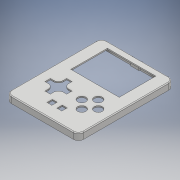
# Autodesk Inventor part: CaseOutline
Saved by Autodesk Inventor 2017 SP1 (Build 210196100, 196)
## iProperties
Created: 2017-08-23
Part Number: CaseOutline
Material: Generic
Document SubType Name: Modeling
Designer: Groguard
Density: 1 g/cm^3
Appearance: Default
Author: Groguard
Autodesk Inventor part; units mm, degrees
ref_plane "YZ Plane" through (0, 0, 0) normal (1, 0, 0) x (0, 1, 0)
ref_plane "XZ Plane" through (0, 0, 0) normal (0, 1, 0) x (-1, 0, 0)
ref_plane "XY Plane" through (0, 0, 0) normal (0, 0, 1) x (1, 0, 0)
sketch "Sketch1" plane through (0, 0, 0) normal (0, 0, 1) x (1, 0, 0)
  line L0 (3.4142, 110) -> (35, 110)
  line L1 (47, 110) -> (78.5858, 110)
  arc A0 (82, 106.5858) -> (78.5858, 110) centre (78.5858, 106.5858) ccw
  arc A1 (47, 110) -> (46, 109) centre (47, 109) ccw
  arc A2 (36, 109) -> (35, 110) centre (35, 109) ccw
  line L2 (36, 109) -> (46, 109)
  arc A3 (3.4142, 110) -> (0, 106.5858) centre (3.4142, 106.5858) ccw
  line L3 (0, 106.5858) -> (0, 3.4142)
  arc A4 (0, 3.4142) -> (3.4142, 0) centre (3.4142, 3.4142) ccw
  arc A5 (78.5858, 0) -> (82, 3.4142) centre (78.5858, 3.4142) ccw
  line L4 (82, 3.4142) -> (82, 106.5858)
  line L5 (3.4142, 0) -> (78.5858, 0)
  line L6 (-3, 3.4142) -> (-3, 106.5858)
  arc A6 (3.4142, 113) -> (-3, 106.5858) centre (3.4142, 106.5858) ccw
  line L7 (3.4142, 113) -> (35, 113)
  arc A7 (37.6458, 112) -> (35, 113) centre (35, 109) ccw
  line L8 (37.6458, 112) -> (44.3542, 112)
  arc A8 (47, 113) -> (44.3542, 112) centre (47, 109) ccw
  line L9 (47, 113) -> (78.5858, 113)
  arc A9 (85, 106.5858) -> (78.5858, 113) centre (78.5858, 106.5858) ccw
  line L10 (85, 106.5858) -> (85, 3.4142)
  arc A10 (78.5858, -3) -> (85, 3.4142) centre (78.5858, 3.4142) ccw
  line L11 (78.5858, -3) -> (3.4142, -3)
  arc A11 (-3, 3.4142) -> (3.4142, -3) centre (3.4142, 3.4142) ccw
  arc A12 (70.4, 61.0119) -> (70.4, 61.0881) centre (70.4, 61.05) ccw
  arc A13 (11.6, 61.0881) -> (11.6, 61.0119) centre (11.6, 61.05) ccw
  line L12 (70.4, 61.05) -> (70.4, 105.55)
  arc A14 (70.4381, 105.55) -> (70.3619, 105.55) centre (70.4, 105.55) ccw
  arc A15 (70.3619, 61.05) -> (70.4381, 61.05) centre (70.4, 61.05) ccw
  arc A16 (11.6, 105.5881) -> (11.6, 105.5119) centre (11.6, 105.55) ccw
  arc A17 (70.4, 105.5119) -> (70.4, 105.5881) centre (70.4, 105.55) ccw
  line L13 (11.6, 105.55) -> (11.6, 61.05)
  arc A18 (11.5619, 61.05) -> (11.6381, 61.05) centre (11.6, 61.05) ccw
  arc A19 (11.6381, 105.55) -> (11.5619, 105.55) centre (11.6, 105.55) ccw
  line L14 (11.6, 61.05) -> (70.4, 61.05)
  arc A20 (30.1856, 85.7097) -> (30.4452, 85.4501) centre (30.4452, 85.7097) ccw
  arc A21 (30.211, 85.7097) -> (30.1602, 85.7097) centre (30.1856, 85.7097) ccw
  arc A22 (30.4452, 85.4247) -> (30.4452, 85.4755) centre (30.4452, 85.4501) ccw
  line L15 (30.1856, 85.7097) -> (30.1856, 85.7746)
  arc A23 (30.211, 85.7746) -> (30.1602, 85.7746) centre (30.1856, 85.7746) ccw
  arc A24 (30.1602, 85.7097) -> (30.211, 85.7097) centre (30.1856, 85.7097) ccw
  arc A25 (30.8347, 85.7746) -> (30.1856, 85.7746) centre (30.5102, 85.7746) ccw
  arc A26 (30.8093, 85.7746) -> (30.8601, 85.7746) centre (30.8347, 85.7746) ccw
  arc A27 (30.1602, 85.7746) -> (30.211, 85.7746) centre (30.1856, 85.7746) ccw
  line L16 (30.8347, 85.7746) -> (30.8347, 85.4501)
  arc A28 (30.8093, 85.4501) -> (30.8601, 85.4501) centre (30.8347, 85.4501) ccw
  arc A29 (30.8601, 85.7746) -> (30.8093, 85.7746) centre (30.8347, 85.7746) ccw
  arc A30 (30.3154, 84.9308) -> (30.8347, 85.4501) centre (30.3154, 85.4501) ccw
  arc A31 (30.3154, 84.9562) -> (30.3154, 84.9054) centre (30.3154, 84.9308) ccw
  arc A32 (30.8601, 85.4501) -> (30.8093, 85.4501) centre (30.8347, 85.4501) ccw
  line L17 (31.3286, 84.9308) -> (31.6531, 84.9308)
  arc A33 (31.6531, 84.9054) -> (31.6531, 84.9562) centre (31.6531, 84.9308) ccw
  arc A34 (31.3286, 84.9562) -> (31.3286, 84.9054) centre (31.3286, 84.9308) ccw
  arc A35 (31.6531, 84.9308) -> (31.6531, 85.5799) centre (31.6531, 85.2553) ccw
  arc A36 (31.6531, 84.9562) -> (31.6531, 84.9054) centre (31.6531, 84.9308) ccw
  arc A37 (31.6531, 85.6053) -> (31.6531, 85.5545) centre (31.6531, 85.5799) ccw
  line L18 (31.3286, 86.0992) -> (31.7181, 86.0992)
  arc A38 (31.7181, 86.0738) -> (31.7181, 86.1246) centre (31.7181, 86.0992) ccw
  arc A39 (31.3286, 86.1246) -> (31.3286, 86.0738) centre (31.3286, 86.0992) ccw
  arc A40 (31.7181, 85.5799) -> (31.7181, 86.0992) centre (31.7181, 85.8396) ccw
  arc A41 (31.7181, 85.6053) -> (31.7181, 85.5545) centre (31.7181, 85.5799) ccw
  arc A42 (31.7181, 86.1246) -> (31.7181, 86.0738) centre (31.7181, 86.0992) ccw
  line L19 (31.7181, 85.5799) -> (31.4584, 85.5799)
  arc A43 (31.4584, 85.6053) -> (31.4584, 85.5545) centre (31.4584, 85.5799) ccw
  arc A44 (31.7181, 85.5545) -> (31.7181, 85.6053) centre (31.7181, 85.5799) ccw
  line L20 (32.7312, 86.0992) -> (32.4716, 85.1904)
  arc A45 (32.4472, 85.1974) -> (32.496, 85.1835) centre (32.4716, 85.1904) ccw
  arc A46 (32.7557, 86.0922) -> (32.7068, 86.1062) centre (32.7313, 86.0992) ccw
  line L21 (32.4716, 85.1904) -> (33.1207, 85.1904)
  arc A47 (33.1207, 85.165) -> (33.1207, 85.2158) centre (33.1207, 85.1904) ccw
  arc A48 (32.4716, 85.2158) -> (32.4716, 85.165) centre (32.4716, 85.1904) ccw
  line L22 (32.926, 85.4501) -> (32.926, 84.9308)
  arc A49 (32.9006, 84.9308) -> (32.9514, 84.9308) centre (32.926, 84.9308) ccw
  arc A50 (32.9514, 85.4501) -> (32.9006, 85.4501) centre (32.926, 85.4501) ccw
  line L23 (33.6146, 85.8396) -> (33.9391, 86.0992)
  arc A51 (33.955, 86.0794) -> (33.9233, 86.119) centre (33.9391, 86.0992) ccw
  arc A52 (33.5987, 85.8594) -> (33.6304, 85.8197) centre (33.6146, 85.8396) ccw
  line L24 (33.9391, 86.0992) -> (33.9391, 84.9308)
  arc A53 (33.9137, 84.9308) -> (33.9645, 84.9308) centre (33.9391, 84.9308) ccw
  arc A54 (33.9645, 86.0992) -> (33.9137, 86.0992) centre (33.9391, 86.0992) ccw
  line L25 (33.6146, 84.9308) -> (34.2637, 84.9308)
  arc A55 (34.2637, 84.9054) -> (34.2637, 84.9562) centre (34.2637, 84.9308) ccw
  arc A56 (33.6146, 84.9562) -> (33.6146, 84.9054) centre (33.6146, 84.9308) ccw
  line L26 (34.7689, 85.3852) -> (35.5478, 85.3852)
  arc A57 (35.5478, 85.3598) -> (35.5478, 85.4106) centre (35.5478, 85.3852) ccw
  arc A58 (34.7689, 85.4106) -> (34.7689, 85.3598) centre (34.7689, 85.3852) ccw
  arc A59 (36.7021, 85.8071) -> (36.41, 86.0992) centre (36.41, 85.8071) ccw
  arc A60 (36.6767, 85.8071) -> (36.7275, 85.8071) centre (36.7021, 85.8071) ccw
  arc A61 (36.41, 86.1246) -> (36.41, 86.0738) centre (36.41, 86.0992) ccw
  arc A62 (36.41, 86.0992) -> (36.053, 85.8396) centre (36.41, 85.724) ccw
  arc A63 (36.41, 86.0738) -> (36.41, 86.1246) centre (36.41, 86.0992) ccw
  arc A64 (36.0288, 85.8474) -> (36.0771, 85.8317) centre (36.0529, 85.8396) ccw
  arc A65 (36.6047, 85.5799) -> (36.7021, 85.8071) centre (36.3884, 85.8071) ccw
  arc A66 (36.5872, 85.5983) -> (36.6222, 85.5615) centre (36.6047, 85.5799) ccw
  arc A67 (36.7275, 85.8071) -> (36.6767, 85.8071) centre (36.7021, 85.8071) ccw
  line L27 (36.6047, 85.5799) -> (36.053, 84.9308)
  arc A68 (36.0336, 84.9473) -> (36.0723, 84.9143) centre (36.0529, 84.9308) ccw
  arc A69 (36.6241, 85.5635) -> (36.5854, 85.5964) centre (36.6047, 85.5799) ccw
  line L28 (36.053, 84.9308) -> (36.7021, 84.9308)
  arc A70 (36.7021, 84.9054) -> (36.7021, 84.9562) centre (36.7021, 84.9308) ccw
  arc A71 (36.053, 84.9562) -> (36.053, 84.9054) centre (36.053, 84.9308) ccw
  arc A72 (37.8451, 85.2554) -> (37.196, 85.2554) centre (37.5206, 85.2554) ccw
  arc A73 (37.8197, 85.2554) -> (37.8705, 85.2554) centre (37.8451, 85.2554) ccw
  arc A74 (37.1706, 85.2554) -> (37.2214, 85.2554) centre (37.196, 85.2554) ccw
  arc A75 (37.196, 85.2554) -> (37.8451, 85.2554) centre (37.5206, 85.2554) ccw
  arc A76 (37.2214, 85.2554) -> (37.1706, 85.2554) centre (37.196, 85.2554) ccw
  arc A77 (37.8705, 85.2554) -> (37.8197, 85.2554) centre (37.8451, 85.2554) ccw
  arc A78 (37.7802, 85.8396) -> (37.2609, 85.8396) centre (37.5206, 85.8396) ccw
  arc A79 (37.7548, 85.8396) -> (37.8056, 85.8396) centre (37.7802, 85.8396) ccw
  arc A80 (37.2355, 85.8396) -> (37.2863, 85.8396) centre (37.2609, 85.8396) ccw
  arc A81 (37.2609, 85.8396) -> (37.7802, 85.8396) centre (37.5206, 85.8396) ccw
  arc A82 (37.2863, 85.8396) -> (37.2355, 85.8396) centre (37.2609, 85.8396) ccw
  arc A83 (37.8056, 85.8396) -> (37.7548, 85.8396) centre (37.7802, 85.8396) ccw
  line L29 (50, 18.25) -> (50, 11.75)
  arc A84 (50.0508, 18.25) -> (49.9492, 18.25) centre (50, 18.25) ccw
  line L30 (50, 11.75) -> (44, 11.75)
  line L31 (44, 11.75) -> (44, 18.25)
  arc A85 (44.0508, 18.25) -> (43.9492, 18.25) centre (44, 18.25) ccw
  line L32 (44, 18.25) -> (50, 18.25)
  arc A86 (50, 18.1992) -> (50, 18.3008) centre (50, 18.25) ccw
  arc A87 (44, 18.3008) -> (44, 18.1992) centre (44, 18.25) ccw
  line L33 (38, 18.25) -> (38, 11.75)
  arc A88 (38.0508, 18.25) -> (37.9492, 18.25) centre (38, 18.25) ccw
  line L34 (38, 11.75) -> (32, 11.75)
  line L35 (32, 11.75) -> (32, 18.25)
  arc A89 (32.0508, 18.25) -> (31.9492, 18.25) centre (32, 18.25) ccw
  line L36 (32, 18.25) -> (38, 18.25)
  arc A90 (38, 18.1992) -> (38, 18.3008) centre (38, 18.25) ccw
  arc A91 (32, 18.3008) -> (32, 18.1992) centre (32, 18.25) ccw
  line L37 (3.96, 108.28) -> (73.16, 108.28)
  arc A92 (73.16, 108.2482) -> (73.16, 108.3118) centre (73.16, 108.28) ccw
  arc A93 (3.96, 108.3118) -> (3.96, 108.2482) centre (3.96, 108.28) ccw
  line L38 (73.16, 108.28) -> (73.16, 58.28)
  arc A94 (73.1282, 58.28) -> (73.1917, 58.28) centre (73.16, 58.28) ccw
  arc A95 (73.1917, 108.28) -> (73.1282, 108.28) centre (73.16, 108.28) ccw
  line L39 (73.16, 58.28) -> (3.96, 58.28)
  arc A96 (3.96, 58.3118) -> (3.96, 58.2482) centre (3.96, 58.28) ccw
  arc A97 (73.16, 58.2482) -> (73.16, 58.3118) centre (73.16, 58.28) ccw
  line L40 (3.96, 58.28) -> (3.96, 108.28)
  arc A98 (3.9918, 108.28) -> (3.9283, 108.28) centre (3.96, 108.28) ccw
  arc A99 (3.9283, 58.28) -> (3.9918, 58.28) centre (3.96, 58.28) ccw
  line L41 (20.6108, 93.6396) -> (20.9354, 93.8992)
  arc A100 (20.9512, 93.8794) -> (20.9195, 93.919) centre (20.9353, 93.8992) ccw
  arc A101 (20.5949, 93.6594) -> (20.6267, 93.6197) centre (20.6108, 93.6396) ccw
  line L42 (20.9354, 93.8992) -> (20.9354, 92.7308)
  arc A102 (20.91, 92.7308) -> (20.9608, 92.7308) centre (20.9354, 92.7308) ccw
  arc A103 (20.9608, 93.8992) -> (20.91, 93.8992) centre (20.9354, 93.8992) ccw
  line L43 (20.6108, 92.7308) -> (21.2599, 92.7308)
  arc A104 (21.2599, 92.7054) -> (21.2599, 92.7562) centre (21.2599, 92.7308) ccw
  arc A105 (20.6108, 92.7562) -> (20.6108, 92.7054) centre (20.6108, 92.7308) ccw
  line L44 (20.6108, 74.2396) -> (20.9354, 74.4992)
  arc A106 (20.9512, 74.4794) -> (20.9195, 74.519) centre (20.9353, 74.4992) ccw
  arc A107 (20.5949, 74.2594) -> (20.6267, 74.2197) centre (20.6108, 74.2396) ccw
  line L45 (20.9354, 74.4992) -> (20.9354, 73.3308)
  arc A108 (20.91, 73.3308) -> (20.9608, 73.3308) centre (20.9354, 73.3308) ccw
  arc A109 (20.9608, 74.4992) -> (20.91, 74.4992) centre (20.9354, 74.4992) ccw
  line L46 (20.6108, 73.3308) -> (21.2599, 73.3308)
  arc A110 (21.2599, 73.3054) -> (21.2599, 73.3562) centre (21.2599, 73.3308) ccw
  arc A111 (20.6108, 73.3562) -> (20.6108, 73.3054) centre (20.6108, 73.3308) ccw
  arc A112 (22.4029, 73.6554) -> (21.7538, 73.6554) centre (22.0784, 73.6554) ccw
  arc A113 (22.3775, 73.6554) -> (22.4283, 73.6554) centre (22.4029, 73.6554) ccw
  arc A114 (21.7284, 73.6554) -> (21.7792, 73.6554) centre (21.7538, 73.6554) ccw
  arc A115 (21.7538, 73.6554) -> (22.4029, 73.6554) centre (22.0784, 73.6554) ccw
  arc A116 (21.7792, 73.6554) -> (21.7284, 73.6554) centre (21.7538, 73.6554) ccw
  arc A117 (22.4283, 73.6554) -> (22.3775, 73.6554) centre (22.4029, 73.6554) ccw
  arc A118 (22.338, 74.2396) -> (21.8187, 74.2396) centre (22.0784, 74.2396) ccw
  arc A119 (22.3126, 74.2396) -> (22.3634, 74.2396) centre (22.338, 74.2396) ccw
  arc A120 (21.7933, 74.2396) -> (21.8441, 74.2396) centre (21.8187, 74.2396) ccw
  arc A121 (21.8187, 74.2396) -> (22.338, 74.2396) centre (22.0784, 74.2396) ccw
  arc A122 (21.8441, 74.2396) -> (21.7933, 74.2396) centre (21.8187, 74.2396) ccw
  arc A123 (22.3634, 74.2396) -> (22.3126, 74.2396) centre (22.338, 74.2396) ccw
  line L47 (28.6433, 84.9308) -> (28.6433, 85.7097)
  arc A124 (28.6687, 85.7097) -> (28.6179, 85.7097) centre (28.6433, 85.7097) ccw
  arc A125 (28.6179, 84.9308) -> (28.6687, 84.9308) centre (28.6433, 84.9308) ccw
  line L48 (28.6108, 86.0343) -> (28.6108, 86.0992)
  arc A126 (28.6362, 86.0992) -> (28.5854, 86.0992) centre (28.6108, 86.0992) ccw
  arc A127 (28.5854, 86.0343) -> (28.6362, 86.0343) centre (28.6108, 86.0343) ccw
  line L49 (28.6108, 86.0992) -> (28.6757, 86.0992)
  arc A128 (28.6757, 86.0738) -> (28.6757, 86.1246) centre (28.6757, 86.0992) ccw
  arc A129 (28.6108, 86.1246) -> (28.6108, 86.0738) centre (28.6108, 86.0992) ccw
  line L50 (28.6757, 86.0992) -> (28.6757, 86.0343)
  arc A130 (28.6503, 86.0343) -> (28.7011, 86.0343) centre (28.6757, 86.0343) ccw
  arc A131 (28.7011, 86.0992) -> (28.6503, 86.0992) centre (28.6757, 86.0992) ccw
  line L51 (28.6757, 86.0343) -> (28.6108, 86.0343)
  arc A132 (28.6108, 86.0597) -> (28.6108, 86.0089) centre (28.6108, 86.0343) ccw
  arc A133 (28.6757, 86.0089) -> (28.6757, 86.0597) centre (28.6757, 86.0343) ccw
  line L52 (29.1225, 86.0992) -> (29.1225, 85.1255)
  arc A134 (29.0971, 85.1255) -> (29.1479, 85.1255) centre (29.1225, 85.1255) ccw
  arc A135 (29.1479, 86.0992) -> (29.0971, 86.0992) centre (29.1225, 86.0992) ccw
  arc A136 (29.1225, 85.1255) -> (29.3172, 84.9308) centre (29.3172, 85.1255) ccw
  arc A137 (29.1479, 85.1255) -> (29.0971, 85.1255) centre (29.1225, 85.1255) ccw
  arc A138 (29.3172, 84.9054) -> (29.3172, 84.9562) centre (29.3172, 84.9308) ccw
  line L53 (29.71, 84.9308) -> (29.71, 85.7097)
  arc A139 (29.7354, 85.7097) -> (29.6846, 85.7097) centre (29.71, 85.7097) ccw
  arc A140 (29.6846, 84.9308) -> (29.7354, 84.9308) centre (29.71, 84.9308) ccw
  line L54 (29.6776, 86.0343) -> (29.6776, 86.0992)
  arc A141 (29.703, 86.0992) -> (29.6522, 86.0992) centre (29.6776, 86.0992) ccw
  arc A142 (29.6522, 86.0343) -> (29.703, 86.0343) centre (29.6776, 86.0343) ccw
  line L55 (29.6776, 86.0992) -> (29.7425, 86.0992)
  arc A143 (29.7425, 86.0738) -> (29.7425, 86.1246) centre (29.7425, 86.0992) ccw
  arc A144 (29.6776, 86.1246) -> (29.6776, 86.0738) centre (29.6776, 86.0992) ccw
  line L56 (29.7425, 86.0992) -> (29.7425, 86.0343)
  arc A145 (29.7171, 86.0343) -> (29.7679, 86.0343) centre (29.7425, 86.0343) ccw
  arc A146 (29.7679, 86.0992) -> (29.7171, 86.0992) centre (29.7425, 86.0992) ccw
  line L57 (29.7425, 86.0343) -> (29.6776, 86.0343)
  arc A147 (29.6776, 86.0597) -> (29.6776, 86.0089) centre (29.6776, 86.0343) ccw
  arc A148 (29.7425, 86.0089) -> (29.7425, 86.0597) centre (29.7425, 86.0343) ccw
  line L58 (30.8347, 85.4501) -> (30.4452, 85.4501)
  arc A149 (30.4452, 85.4755) -> (30.4452, 85.4247) centre (30.4452, 85.4501) ccw
  arc A150 (30.8347, 85.4247) -> (30.8347, 85.4755) centre (30.8347, 85.4501) ccw
  line L59 (70.4, 105.55) -> (70.4, 61.05)
  line L60 (32, 18.25) -> (38, 18.25)
  line L61 (38, 18.25) -> (38, 11.75)
  line L62 (38, 11.75) -> (32, 11.75)
  line L63 (32, 11.75) -> (32, 18.25)
  line L64 (44, 18.25) -> (50, 18.25)
  line L65 (50, 18.25) -> (50, 11.75)
  line L66 (50, 11.75) -> (44, 11.75)
  line L67 (44, 11.75) -> (44, 18.25)
  circle A151 centre (60, 46) radius 5
  circle A152 centre (50, 36) radius 5
  circle A153 centre (60, 26) radius 5
  circle A154 centre (70, 36) radius 5
  line L68 (70.4, 105.55) -> (11.6, 105.55)
  line L69 (11.6, 105.55) -> (11.6, 61.05)
  line L70 (11.6, 61.05) -> (70.4, 61.05)
  line L71 (31.25, 39) -> (35.25, 39)
  line L72 (35.25, 39) -> (35.25, 32.5)
  line L73 (35.25, 32.5) -> (31.25, 32.5)
  line L74 (25.25, 26.5) -> (25.25, 22.5)
  line L75 (25.25, 45) -> (25.25, 49)
  line L76 (25.25, 49) -> (18.75, 49)
  line L77 (18.75, 49) -> (18.75, 45)
  line L78 (12.75, 39) -> (8.75, 39)
  line L79 (8.75, 39) -> (8.75, 32.5)
  line L80 (8.75, 32.5) -> (12.75, 32.5)
  line L81 (18.75, 26.5) -> (18.75, 22.5)
  line L82 (18.75, 22.5) -> (25.25, 22.5)
  arc A155 (12.75, 39) -> (18.75, 45) centre (12.75, 45) ccw
  arc A156 (25.25, 45) -> (31.25, 39) centre (31.25, 45) ccw
  arc A157 (31.25, 32.5) -> (25.25, 26.5) centre (31.25, 26.5) ccw
  arc A158 (18.75, 26.5) -> (12.75, 32.5) centre (12.75, 26.5) ccw
  point P0 (0, 0)
  point P1 (18.75, 39)
  point P2 (18.75, 32.5)
  dimension "d0" = 3
  dimension "d1" = 10
  dimension "d2" = 10
  dimension "d3" = 10
  dimension "d4" = 10
  dimension "d12" = 6.5
  dimension "d13" = 10
  dimension "d18" = 6
  constraints: 310 point on circle, 166 end point, 159 centre point, 10 perpendicular, 8 tangent, 6 point on line, 5 horizontal, 4 parallel, 3 equal radius, 2 vertical, 11 other
  measures "d0" distance between parallel lines of L3 L6
  measures "d1" diameter of A151
  measures "d2" diameter of A152
  measures "d3" diameter of A153
  measures "d4" diameter of A154
  measures "d12" distance of L75.end L76.end
  measures "d13" distance of L76.end point (18.75, 39)
  measures "d18" radius of A155
extrude "Extrusion1" add sketch "Sketch1" along normal blind 1.5 contours L0 A2 L2 A1 L1 A0 L4 A5 L5 A4 L3 A3 | L6 A6 L7 A7 L8 A8 L9 A9 L10 A10 L11 A11 | A15 L14 L12 A12 | A18 A13 L13 L14 | L12 L68 A14 A17 | A16 A19 L68 L13 | L32 A84 A86 L29 | L32 L31 A87 A85 | L36 A88 A90 L33 | L36 L35 A91 A89 | L40 A93 A98 L37 | L37 L38 L39 L40 | A95 A92 L38 L37 | L40 L39 A99 A96 | A97 A94 L39 L38
sketch "Sketch2" plane through (0, 0, 0) normal (0, 0, -1) x (-1, 0, 0)
  arc A0 (-78.5858, 113) -> (-85, 106.5858) centre (-78.5858, 106.5858) ccw projected
  line L0 (-85, 106.5858) -> (-85, 3.4142) projected
  line L1 (-85, 106.5858) -> (-85, 3.4142)
  arc A1 (-85, 3.4142) -> (-78.5858, -3) centre (-78.5858, 3.4142) ccw projected
  arc A2 (-85, 3.4142) -> (-85, 3.4142) centre (-78.5858, 3.4142) ccw
  line L2 (-3.4142, -3) -> (-78.5858, -3) projected
  line L3 (-78.5858, -3) -> (-3.4142, -3)
  line L4 (-47, 113) -> (-78.5858, 113) projected
  line L5 (-78.5858, 113) -> (-47, 113)
  arc A3 (-44.3542, 112) -> (-47, 113) centre (-47, 109) ccw projected
  arc A4 (-47, 113) -> (-47, 113) centre (-47, 109) ccw
  line L6 (-37.6458, 112) -> (-44.3542, 112) projected
  line L7 (-44.3542, 112) -> (-37.6458, 112)
  arc A5 (-35, 113) -> (-37.6458, 112) centre (-35, 109) ccw projected
  arc A6 (-37.6458, 112) -> (-37.6458, 112) centre (-35, 109) ccw
  line L8 (-35, 113) -> (-3.4142, 113) projected
  line L9 (-35, 113) -> (-3.4142, 113)
  arc A7 (3, 106.5858) -> (-3.4142, 113) centre (-3.4142, 106.5858) ccw projected
  arc A8 (3, 106.5858) -> (-3.4142, 113) centre (-3.4142, 106.5858) ccw
  line L10 (3, 3.4142) -> (3, 106.5858) projected
  line L11 (3, 106.5858) -> (3, 3.4142)
  arc A9 (-3.4142, -3) -> (3, 3.4142) centre (-3.4142, 3.4142) ccw projected
  arc A10 (3, 3.4142) -> (3, 3.4142) centre (-3.4142, 3.4142) ccw
  arc A11 (-78.5858, 110) -> (-82, 106.5858) centre (-78.5858, 106.5858) ccw
  line L12 (-82, 106.5858) -> (-82, 3.4142)
  arc A12 (-82, 3.4142) -> (-78.5858, 0) centre (-78.5858, 3.4142) ccw
  line L13 (-78.5858, 0) -> (-3.4142, 0)
  arc A13 (-3.4142, 0) -> (0, 3.4142) centre (-3.4142, 3.4142) ccw
  line L14 (0, 3.4142) -> (0, 106.5858)
  arc A14 (0, 106.5858) -> (-3.4142, 110) centre (-3.4142, 106.5858) ccw
  line L15 (-3.4142, 110) -> (-35, 110)
  arc A15 (-35, 110) -> (-36, 109) centre (-35, 109) ccw
  line L16 (-36, 109) -> (-46, 109)
  arc A16 (-46, 109) -> (-47, 110) centre (-47, 109) ccw
  line L17 (-47, 110) -> (-78.5858, 110)
  point P0 (0, 0)
  dimension "d21" = 3
  constraints: 24 end point, 14 point on circle, 7 centre point, 6 collinear, 2 horizontal alignment, 1 vertical alignment, 24 other
  measures "d21" distance between parallel lines of L4 L17
extrude "Extrusion2" add sketch "Sketch2" along normal blind 6.5 contours L4 A4 L17 A11 L12 A2 L0 A0 | A3 A4 L16 A16 L17 | A2 L12 A12 L13 A1 | L6 A6 L16 A4 | A2 L13 A10 L2 | A5 A6 L15 A15 L16 | A10 L13 A13 L14 A9 | L8 A7 L10 A10 L14 A14 L15 A6
fillet "Fillet1" radius 1 11 edges at (-1.1213, -1.1213, 1.5) (41, -3, 1.5) (83.1213, -1.1213, 1.5) (85, 55, 1.5) (83.1213, 111.1213, 1.5) (62.7929, 113, 1.5) (45.5858, 112.7417, 1.5) (-1.1213, 111.1213, 1.5) (19.2071, 113, 1.5) (36.4142, 112.7417, 1.5) (-3, 55, 1.5)
body "Solid1"
